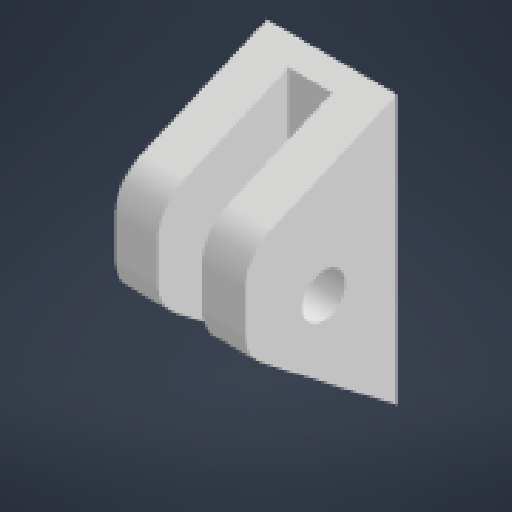
# Autodesk Inventor part: LeverHolder
Saved by Autodesk Inventor 2024.1 (Build 281209000, 209)
## iProperties
Created: 2023-08-22
Part Number: LeverHolder
Material: Generic
Document SubType Name: Modeling
Designer: Eleanor
Density: 1 g/cm^3
Appearance: Default
Author: Eleanor
Autodesk Inventor part; units mm, degrees
ref_plane "YZ Plane" through (0, 0, 0) normal (1, 0, 0) x (0, 1, 0)
ref_plane "XZ Plane" through (0, 0, 0) normal (0, 1, 0) x (-1, 0, 0)
ref_plane "XY Plane" through (0, 0, 0) normal (0, 0, 1) x (1, 0, 0)
sketch "Sketch1" plane through (0, 0, 0) normal (1, 0, 0) x (0, 1, 0)
  line L0 (-9.6115, 8.22) -> (-14.9205, 8.22)
  line L1 (-14.9205, 8.22) -> (-21.231, 0)
  line L2 (-21.231, 0) -> (-1.5875, 0)
  line L3 (-9.6115, 8.22) -> (-8.1578, 3.0283)
  line L4 (-8.1578, 3.0283) -> (-1.5875, 0)
  point P0 (0, 0)
  constraints: 10 end point, 1 horizontal, 1 parallel
extrude "Extrusion1" add sketch "Sketch1" along normal blind 9.525
fillet "Fillet1" radius 3.175 2 edges at (4.7625, -9.6115, 8.22) (4.7625, -14.9205, 8.22)
sketch "Sketch3" plane through (0, -13.3553, 8.22) normal (0, 0, 1) x (1, 0, 0)
  line L0 (6.35, -11.8558) -> (6.35, 11.9002)
  line L1 (6.35, 11.9002) -> (3.175, 11.9002)
  line L2 (3.175, 11.9002) -> (3.175, -11.8558)
  line L3 (3.175, -11.8558) -> (6.35, -11.8558)
  line L4 (0, 0.0222) -> (9.525, 0.0222) projected
  line L5 (6.35, -11.8558) -> (3.175, 11.9002) construction
  line L6 (6.35, 11.9002) -> (3.175, -11.8558) construction
  point P0 (0, 13.3553)
  point P1 (4.7625, 0.0222)
  constraints: 12 end point, 3 midpoint, 2 parallel, 2 perpendicular
extrude "Extrusion2" cut sketch "Sketch3" against normal blind 9.525
sketch "Sketch4" plane through (0, 0, 0) normal (-1, 0, 0) x (0, 0, 1)
  circle A0 centre (5.3647, -11.6366) radius 1.5875
  point P0 (0, 0)
  constraints: 1 centre point
extrude "Extrusion3" cut sketch "Sketch4" against normal blind 9.525
fillet "Fillet2" radius 3.175 2 edges at (1.5875, -8.1578, 3.0283) (7.9375, -8.1578, 3.0283)
body "Solid1"
